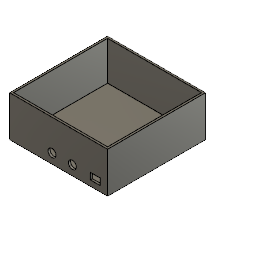
Case (Autodesk Fusion 360 design; units mm, degrees)
Autodesk Fusion 360 part; units mm, degrees
sketch "Sketch1" plane through (0, 0, 0) normal (0, 1, 0) x (1, 0, 0)
  line L0 (0, 0) -> (120, 0)
  line L1 (120, 0) -> (120, -120)
  line L2 (120, -120) -> (0, -120)
  line L3 (0, -120) -> (0, 0)
  dimension "d1" = 120
  dimension "d2" = 120
  constraint horizontal L0
  constraint vertical L1
  constraint horizontal L2
  constraint vertical L3
  constraint coincident L0.start L3.end
  measures "d1" distance of L0.start L0.end
  measures "d2" distance of L0.start L2.end
extrude "Extrude1" add sketch "Sketch1" along normal blind 50
sketch "Sketch2" plane through (0, 50, 0) normal (0, 1, 0) x (-1, 0, 0)
  line L0 (0, 120) -> (-120, 120)
  line L1 (-120, 120) -> (-120, 0)
  line L2 (-120, 0) -> (0, 0)
  line L3 (0, 0) -> (0, 120)
  line L4 (-2.5, 2.5) -> (-117.5, 2.5)
  line L5 (-117.5, 2.5) -> (-117.5, 117.5)
  line L6 (-117.5, 117.5) -> (-2.5, 117.5)
  line L7 (-2.5, 117.5) -> (-2.5, 2.5)
  dimension "d5" = 115
  dimension "d6" = 115
  dimension "d7" = 2.5
  dimension "d8" = 2.5
  constraint horizontal L4
  constraint vertical L5
  constraint horizontal L6
  constraint vertical L7
  measures "d5" distance of L4.start L4.end
  measures "d6" distance of L4.start L6.end
  measures "d7" distance of L2 L4
  measures "d8" distance of L3 L7
extrude "Extrude2" cut sketch "Sketch2" against normal blind 47.5 contours L4 L5 L6 L7
move_body "Align1" bodies 1 to x (1, 0, 0) y (0, 1, 0) z (0, 0, 1) at (0, 0, 0)
sketch "Sketch3" plane through (0, 0, 120) normal (0, 0, 1) x (1, 0, 0)
  line L0 (0, 0) -> (120, 0)
  line L1 (120, 0) -> (120, 50)
  line L2 (120, 50) -> (0, 50)
  line L3 (0, 50) -> (0, 0)
  circle A0 centre (77, 12) radius 4.85
  circle A1 centre (52, 12) radius 4.85
  line L4 (99, 15) -> (111, 15)
  line L5 (111, 15) -> (111, 7)
  line L6 (111, 7) -> (99, 7)
  line L7 (99, 7) -> (99, 15)
  dimension "d31" = 12
  dimension "d32" = 8
  dimension "d33" = 9.7
  dimension "d34" = 9.7
  dimension "d35" = 12
  dimension "d36" = 12
  dimension "d37" = 7
  dimension "d38" = 25
  dimension "d39" = 22
  constraint horizontal L4
  constraint vertical L5
  constraint horizontal L6
  constraint vertical L7
  measures "d31" distance of L4.start L4.end
  measures "d32" distance of L4.end L5.end
  measures "d33" diameter of A0
  measures "d34" diameter of A1
  measures "d35" distance of L0 A0.centre
  measures "d36" distance of L0 A1.centre
  measures "d37" distance of L0 L6
  measures "d38" distance of A0.centre A1.centre
  measures "d39" distance of A0.centre L7
extrude "Extrude3" cut sketch "Sketch3" against normal up to surface (2.5 mm away) contours A0 | A1 | L4 L5 L6 L7
